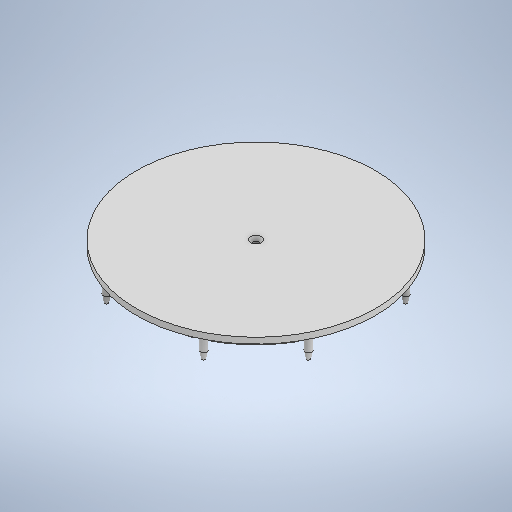
# Autodesk Inventor part: lid
Saved by Autodesk Inventor 2025 (Build 290162000, 162)
## iProperties
Created: 2026-05-09
Part Number: lid
Material: Generic
Document SubType Name: Modeling
Designer: Luca
Density: 1 g/cm^3
Appearance: Default
Author: Luca
Autodesk Inventor part; units mm, degrees
ref_plane "YZ Plane" through (0, 0, 0) normal (1, 0, 0) x (0, 1, 0)
ref_plane "XZ Plane" through (0, 0, 0) normal (0, 1, 0) x (-1, 0, 0)
ref_plane "XY Plane" through (0, 0, 0) normal (0, 0, 1) x (1, 0, 0)
sketch "lid" plane through (0, 0, 0) normal (0, 1, 0) x (-1, 0, 0)
  line L0 (35, 35) -> (-68.5857, 35)
  line L1 (38, 38) -> (-69.4029, 38)
  line L2 (80, 0) -> (-80, 0) construction
  circle A0 centre (0, 0) radius 80
  line L3 (0, -80) -> (0, 80) construction
  line L4 (38, -69.4029) -> (38, 38)
  line L5 (35, -68.5857) -> (35, 35)
  line L6 (0, 0) -> (56.5685, 56.5685) construction
  line L7 (36.5, 36.5) -> (36.5, -71.1881) construction
  line L8 (36.5, 36.5) -> (-71.1881, 36.5) construction
  line L9 (38, 38) -> (35, 35) construction
  line L10 (36.625, -71.1239) -> (36.625, 36.625)
  line L11 (36.375, 36.375) -> (36.375, -71.2521)
  line L12 (38, -69.4029) -> (38, -70.3989)
  line L13 (35, -68.5857) -> (35, -71.9375)
  line L14 (36.375, 36.375) -> (-71.2521, 36.375)
  line L15 (-71.1239, 36.625) -> (36.625, 36.625)
  line L16 (-69.4029, 38) -> (-70.3989, 38)
  line L17 (-68.5857, 35) -> (-71.9375, 35)
  line L18 (35, 34.8232) -> (56.6569, 56.4801)
  line L19 (32.8787, 35) -> (55.4979, 57.6193)
  line L20 (34.8232, 35) -> (56.4801, 56.6569)
  line L21 (35, 32.8787) -> (57.6193, 55.4979)
  line L22 (37.75, 37.75) -> (37.75, -70.5332)
  line L23 (35.25, -71.8153) -> (35.25, 35.25)
  line L24 (37.75, 37.75) -> (-70.5332, 37.75)
  line L25 (-71.8153, 35.25) -> (35.25, 35.25)
  line L26 (33.2322, 35) -> (55.6778, 57.4455)
  line L27 (57.4455, 55.6778) -> (35, 33.2322)
extrude "Extrusion1" add sketch "lid" along normal up to surface (4 mm away) from surface at 0
sketch "reservoir_lid_seal" plane through (0, 0, 0) normal (0, 1, 0) x (-1, 0, 0)
  line L0 (35, -68.5857) -> (35, 35) construction
  line L1 (35.25, -71.8153) -> (35.25, 35.25) construction
  line L2 (36.375, 36.375) -> (36.375, -71.2521) construction
  line L3 (36.5, 36.5) -> (36.5, -71.1881) construction
  line L4 (36.625, -71.1239) -> (36.625, 36.625) construction
  line L5 (37.75, 37.75) -> (37.75, -70.5332) construction
  line L6 (38, -69.4029) -> (38, 38) construction
  line L7 (0, -80) -> (0, 80) construction
  line L8 (80, 0) -> (-80, 0) construction
  line L9 (35, 35) -> (-68.5857, 35) construction
  line L10 (38, 38) -> (-69.4029, 38) construction
  line L11 (38, -69.4029) -> (38, -70.3989) construction
  line L12 (35, -68.5857) -> (35, -71.9375) construction
  line L13 (37.75, 37.75) -> (-70.5332, 37.75) construction
  line L14 (-71.1239, 36.625) -> (36.625, 36.625) construction
  line L15 (36.5, 36.5) -> (-71.1881, 36.5) construction
  line L16 (36.375, 36.375) -> (-71.2521, 36.375) construction
  line L17 (-71.8153, 35.25) -> (35.25, 35.25) construction
  line L18 (-69.4029, 38) -> (-70.3989, 38) construction
  line L19 (-68.5857, 35) -> (-71.9375, 35) construction
  line L20 (0, 0) -> (56.5685, 56.5685) construction
  line L21 (38, 38) -> (35, 35) construction
  line L22 (32.8787, 35) -> (55.4979, 57.6193)
  line L23 (33.2322, 35) -> (55.6778, 57.4455) construction
  line L24 (34.8232, 35) -> (56.4801, 56.6569) construction
  line L25 (35, 34.8232) -> (56.6569, 56.4801) construction
  line L26 (57.4455, 55.6778) -> (35, 33.2322) construction
  line L27 (35, 32.8787) -> (57.6193, 55.4979)
  circle A0 centre (-67.5925, 32.5) radius 2.2 construction
  circle A1 centre (-67.5925, 32.5) radius 2.5 construction
  circle A2 centre (-67.5925, 32.5) radius 5 construction
  line L28 (-67.5925, 32.5) -> (-67.5925, -32.5) construction
  circle A3 centre (-67.5925, -32.5) radius 2.2 construction
  circle A4 centre (-67.5925, -32.5) radius 2.5 construction
  circle A5 centre (-67.5925, -32.5) radius 5 construction
  line L29 (35, 35) -> (-68.5857, 35) construction
  line L30 (38, 38) -> (-69.4029, 38) construction
  circle A6 centre (-32.5, -67.5925) radius 5 construction
  line L31 (35, -68.5857) -> (35, 35) construction
  line L32 (38, -69.4029) -> (38, 38) construction
  circle A7 centre (0, 0) radius 80 construction
  line L33 (-32.5, -67.5925) -> (32.5, -67.5925) construction
  circle A8 centre (32.5, -67.5925) radius 5 construction
  circle A9 centre (-32.5, 67.5925) radius 2.2 construction
  circle A10 centre (-32.5, 67.5925) radius 2.5 construction
  circle A11 centre (67.5925, -32.5) radius 5 construction
  circle A12 centre (67.5925, 32.5) radius 2.2 construction
  circle A13 centre (67.5925, 32.5) radius 2.5 construction
  circle A14 centre (67.5925, 32.5) radius 5 construction
  line L34 (67.5925, 32.5) -> (67.5925, -32.5) construction
  circle A15 centre (67.5925, -32.5) radius 2.2 construction
  circle A16 centre (67.5925, -32.5) radius 2.5 construction
  circle A17 centre (-32.5, 67.5925) radius 5 construction
  circle A18 centre (32.5, 67.5925) radius 2.5 construction
  circle A19 centre (32.5, 67.5925) radius 5 construction
  line L35 (0, 67.5925) -> (0, 0) construction
  circle A20 centre (32.5, 67.5925) radius 2.2 construction
  line L36 (33.7759, 70.2462) -> (34.6667, 72.0987) construction
  line L37 (32.5, 67.5925) -> (-32.5, 67.5925) construction
  circle A21 centre (32.5, -67.5925) radius 2.5 construction
  circle A22 centre (-32.5, -67.5925) radius 2.5 construction
  circle A23 centre (32.5, -67.5925) radius 2.2 construction
  circle A24 centre (-32.5, -67.5925) radius 2.2 construction
  line L38 (67.5925, 0) -> (0, 0) construction
  line L39 (3.4, 0) -> (1.7, -2.9445) construction
  line L40 (1.7, 2.9445) -> (3.4, 0) construction
  line L41 (1.7, -2.9445) -> (-1.7, -2.9445) construction
  circle A25 centre (0, 0) radius 1.35 construction
  circle A26 centre (0, 0) radius 1.6 construction
  line L42 (-1.7, 2.9445) -> (1.7, 2.9445) construction
  line L43 (-1.7, -2.9445) -> (-3.4, 0) construction
  line L44 (-3.4, 0) -> (-1.7, 2.9445) construction
  circle A27 centre (0, 0) radius 5 construction
  circle A28 centre (67.5925, -32.5) radius 5.25
  circle A29 centre (32.5, -67.5925) radius 5.25
  circle A30 centre (-32.5, -67.5925) radius 5.25
  circle A31 centre (-67.5925, -32.5) radius 5.25
  circle A32 centre (-67.5925, 32.5) radius 5.25
  circle A33 centre (-32.5, 67.5925) radius 5.25
  circle A34 centre (32.5, 67.5925) radius 5.25
  circle A35 centre (67.5925, 32.5) radius 5.25
  circle A36 centre (0, 0) radius 5.25
  circle A37 centre (67.5925, -32.5) radius 6.25
  circle A38 centre (67.5925, 32.5) radius 6.25
  circle A39 centre (32.5, 67.5925) radius 6.25
  circle A40 centre (-32.5, 67.5925) radius 6.25
  circle A41 centre (-67.5925, 32.5) radius 6.25
  circle A42 centre (0, 0) radius 6.25
  circle A43 centre (-67.5925, -32.5) radius 6.25
  circle A44 centre (-32.5, -67.5925) radius 6.25
  circle A45 centre (32.5, -67.5925) radius 6.25
  line L45 (34.75, -72.0586) -> (34.75, 34.75)
  line L46 (34.75, 34.75) -> (-68.4324, 34.75)
  line L47 (-67.8159, 33.75) -> (33.75, 33.75)
  line L48 (33.75, 33.75) -> (33.75, -72.5323)
  arc A46 (38.25, -67.9775) -> (-67.9775, 38.25) centre (0, 0) ccw construction
  arc A47 (-68.5857, 35) -> (35, -68.5857) centre (0, 0) ccw construction
  arc A48 (-66.3253, 38.6202) -> (34.75, -68.4324) centre (0, 0) ccw
  arc A49 (-65.3373, 38.3289) -> (33.75, -67.8159) centre (0, 0) ccw
  arc A50 (38.25, -67.6905) -> (-67.6905, 38.25) centre (0, 0) ccw
  arc A51 (39.25, -65.9545) -> (-65.9545, 39.25) centre (0, 0) ccw
  line L49 (38.25, -67.6905) -> (38.25, 38.25)
  line L50 (38.25, 38.25) -> (-67.6905, 38.25)
  line L51 (-65.9545, 39.25) -> (39.25, 39.25)
  line L52 (39.25, 39.25) -> (39.25, -65.9545)
  point P0 (-67.5925, 0)
  point P1 (0, -67.5925)
  point P2 (-61.4688, 33.75)
  point P3 (33.75, -61.4688)
  point P4 (27.0986, -70.737)
  point P5 (-27.0986, -70.737)
  point P6 (-38.3289, -65.3373)
  point P7 (-65.3373, -38.3289)
  point P8 (-70.737, -27.0986)
  point P9 (-70.737, 27.0986)
  point P10 (-62.8491, 34.75)
  point P11 (-71.1911, 28.6773)
  point P12 (-71.1911, -28.6773)
  point P13 (-66.8539, -37.6978)
  point P14 (-37.6978, -66.8539)
  point P15 (-28.6773, -71.1911)
  point P16 (28.6773, -71.1911)
  point P17 (34.75, -62.8491)
  point P18 (37.7358, 67.9785)
  point P19 (29.532, 71.923)
  point P20 (-29.532, 71.923)
  point P21 (-37.7358, 67.9785)
  point P22 (-67.4071, 38.7472)
  point P23 (-65.143, 38.25)
  point P24 (67.9785, -37.7358)
  point P25 (71.923, -29.532)
  point P26 (71.923, 29.532)
  point P27 (67.9785, 37.7358)
  point P28 (66.3253, 38.6202)
  point P29 (71.5815, 27.6885)
  point P30 (71.5815, -27.6885)
  point P31 (66.3253, -38.6202)
  point P32 (-38.6202, 66.3253)
  point P33 (-27.6885, 71.5815)
  point P34 (27.6885, 71.5815)
  point P35 (38.6202, 66.3253)
extrude "Extrusion2" add sketch "reservoir_lid_seal" against normal blind 2 contours L50 A41 A50 A40 A51 L51 L22 | L22 L51 L52 L27 L49 L50 | A51 A39 A50 L22 | L22 A50 L27 A51 | L27 L52 A51 A37 A50 A45 L49 | L46 L45 A45 L48 L47 A41 | A41 L47 A32 L46 | L27 A50 A38 A51 | A51 A34 A50 A39 | A39 A51 A34 | A51 A33 A40 | A40 A50 A33 A51 | A45 A50 L49 | A41 A49 A32 L47 | A51 A35 A38 | A38 A50 A35 A51 | A51 A40 A50 A39 | A39 A50 A34 A51 | L45 A29 L48 A45 | A51 A35 A50 A38 | A38 A50 A37 A51 | A51 A33 A50 A40 | A51 A28 A50 A37 | A37 A51 A28 | L48 A29 A49 A45 | A49 A43 A48 A41 | A41 A48 A32 A49 | A37 A50 A28 A51 | A48 A44 A49 A45 | A45 A49 A29 A48 | A49 A31 A48 A43 | A43 A49 A31 | A48 A30 A49 A44 | A49 A30 A44 | A48 A31 A49 A43 | A43 A49 A44 A48 | A44 A49 A30 A48 | A42
sketch "lid_mount" plane through (0, -70, 0) normal (0, 1, 0) x (-1, 0, 0)
  line L0 (35, -68.5857) -> (35, 35) construction
  line L1 (35, 35) -> (-68.5857, 35) construction
  line L2 (38, 38) -> (-69.4029, 38) construction
  line L3 (38, -69.4029) -> (38, 38) construction
  circle A0 centre (32.5, -67.5925) radius 5
  circle A1 centre (-67.5925, 32.5) radius 5
  circle A2 centre (-67.5925, -32.5) radius 5
  circle A3 centre (-32.5, -67.5925) radius 5
  line L4 (-32.5, -67.5925) -> (32.5, -67.5925) construction
  circle A4 centre (0, 0) radius 80
  circle A5 centre (-67.5925, -32.5) radius 2.5
  circle A6 centre (32.5, -67.5925) radius 2.5
  circle A7 centre (-67.5925, 32.5) radius 2.5
  circle A8 centre (-32.5, -67.5925) radius 2.5
  circle A9 centre (67.5925, -32.5) radius 5
  circle A10 centre (-32.5, 67.5925) radius 5
  circle A11 centre (67.5925, -32.5) radius 2.5
  circle A12 centre (-32.5, 67.5925) radius 2.5
  circle A13 centre (32.5, 67.5925) radius 2.5
  circle A14 centre (32.5, 67.5925) radius 5
  circle A15 centre (67.5925, 32.5) radius 2.5
  circle A16 centre (67.5925, 32.5) radius 5
  line L5 (67.5925, 32.5) -> (67.5925, -32.5) construction
  line L6 (32.5, 67.5925) -> (-32.5, 67.5925) construction
  line L7 (0, 67.5925) -> (0, 0)
  line L8 (67.5925, 0) -> (0, 0)
  circle A17 centre (-67.5925, -32.5) radius 2.2
  circle A18 centre (32.5, 67.5925) radius 2.2
  circle A19 centre (67.5925, 32.5) radius 2.2
  circle A20 centre (32.5, -67.5925) radius 2.2
  circle A21 centre (-32.5, -67.5925) radius 2.2
  circle A22 centre (-67.5925, 32.5) radius 2.2
  circle A23 centre (-32.5, 67.5925) radius 2.2
  line L9 (33.7759, 70.2462) -> (34.6667, 72.0987) construction
  circle A24 centre (67.5925, -32.5) radius 2.2
  circle A25 centre (0, 0) radius 1.6
  line L10 (-3.4, 0) -> (-1.7, 2.9445)
  line L11 (-1.7, 2.9445) -> (1.7, 2.9445)
  line L12 (1.7, 2.9445) -> (3.4, 0)
  line L13 (3.4, 0) -> (1.7, -2.9445)
  line L14 (1.7, -2.9445) -> (-1.7, -2.9445)
  line L15 (-1.7, -2.9445) -> (-3.4, 0)
  circle A26 centre (0, 0) radius 5
  circle A27 centre (0, 0) radius 1.35
  line L16 (-67.5925, 32.5) -> (-67.5925, -32.5) construction
  point P0 (0, -67.5925)
  point P1 (-67.5925, 0)
extrude "Extrusion3" cut sketch "lid_mount" along normal through all contours A25 L8 A27 L7 | L7 A27 L8 A25 | A27 L8 L7 | L7 L8 A27
extrude "Extrusion4" add sketch "lid_mount" against normal blind 15 from surface at 70 contours A17 | A18 | A19 | A20 | A21 | A22 | A23 | A24
chamfer "Chamfer1" distance 1 distance2 5 1 edges at (34.7, -15, 67.5925) measured on face at (34.2, -15, 67.5925)
chamfer "Chamfer2" distance 1 distance2 5 1 edges at (-30.3, -15, 67.5925) measured on face at (-30.8, -15, 67.5925)
chamfer "Chamfer3" distance 1 distance2 5 1 edges at (-65.3925, -15, 32.5) measured on face at (-65.8925, -15, 32.5)
chamfer "Chamfer4" distance 1 distance2 5 1 edges at (-65.3925, -15, -32.5) measured on face at (-65.8925, -15, -32.5)
chamfer "Chamfer5" distance 1 distance2 5 1 edges at (-30.3, -15, -67.5925) measured on face at (-30.8, -15, -67.5925)
chamfer "Chamfer6" distance 1 distance2 5 1 edges at (34.7, -15, -67.5925) measured on face at (34.2, -15, -67.5925)
chamfer "Chamfer7" distance 1 distance2 5 1 edges at (69.7925, -15, -32.5) measured on face at (69.2925, -15, -32.5)
chamfer "Chamfer8" distance 1 distance2 5 1 edges at (69.7925, -15, 32.5) measured on face at (69.2925, -15, 32.5)
sketch "pipe_out" plane through (-77.5, 0, 0) normal (1, 0, 0) x (0, 1, 0)
  line L0 (-132, 0) -> (302, 0)
  circle A0 centre (-10, 0) radius 7.5
  line L1 (0, 153.4424) -> (0, -148.4939)
  circle A1 centre (-10, 0) radius 7.25
  circle A2 centre (-10, 0) radius 5
  circle A3 centre (-10, 0) radius 9.5
  circle A4 centre (-10, 0) radius 6
  circle A5 centre (-10, 0) radius 6.25
  circle A6 centre (-10, 0) radius 9.75
  point P0 (0, 0)
  point P1 (-2.5, 0)
  point P2 (-2.75, 0)
extrude "Extrusion5" cut sketch "pipe_out" along normal mid plane 10
sketch "battery_lid" plane through (0, -57.9, 0) normal (0, 1, 0) x (-1, 0, 0)
  arc A0 (38.25, -67.9775) -> (-67.9775, 38.25) centre (0, 0) ccw construction
  line L0 (0, -80) -> (0, 80) construction
  circle A1 centre (0, 0) radius 80
  arc A2 (-14.9031, 77.5816) -> (-20.7481, 76.2267) centre (0, 0) ccw
  arc A3 (-14.2257, 74.659) -> (-20.0707, 73.3042) centre (0, 0) ccw
  line L1 (-17.1615, 74.0393) -> (-17.8385, 76.9597) construction
  line L2 (-14.9031, 77.5816) -> (-14.2257, 74.659)
  line L3 (-20.0707, 73.3042) -> (-20.7481, 76.2267)
  arc A4 (20.2646, 72.9914) -> (-20.2646, 72.9914) centre (0, 0) ccw
  line L4 (20.2646, 72.9914) -> (21.4009, 77.0844) construction
  line L5 (-20.2646, 72.9914) -> (-21.4009, 77.0844) construction
  line L6 (-14.5278, 74.8555) -> (-15.0922, 77.2903)
  line L7 (-19.8858, 73.6136) -> (-20.4501, 76.0484)
  arc A5 (-14.5278, 74.8555) -> (-19.8858, 73.6136) centre (0, 0) ccw
  arc A6 (-15.0922, 77.2903) -> (-20.4501, 76.0484) centre (0, 0) ccw
  line L8 (25, 80) -> (-25, 80) construction
  line L9 (14.5278, 74.8555) -> (15.0922, 77.2903)
  arc A7 (20.4501, 76.0484) -> (15.0922, 77.2903) centre (0, 0) ccw
  line L10 (19.8858, 73.6136) -> (20.4501, 76.0484)
  arc A8 (19.8858, 73.6136) -> (14.5278, 74.8555) centre (0, 0) ccw
  arc A9 (20.7481, 76.2267) -> (14.9031, 77.5816) centre (0, 0) ccw
  line L11 (17.1615, 74.0393) -> (17.8385, 76.9597) construction
  arc A10 (20.0707, 73.3042) -> (14.2257, 74.659) centre (0, 0) ccw
  line L12 (20.0707, 73.3042) -> (20.7481, 76.2267)
  line L13 (14.9031, 77.5816) -> (14.2257, 74.659)
  line L14 (-27.5, 72.9914) -> (-20.2646, 72.9914)
  line L15 (20.2646, 72.9914) -> (27.5, 72.9914)
  arc A11 (-4.983, 75.5882) -> (4.983, 75.5882) centre (0, 76) ccw
  circle A12 centre (0, 76) radius 3
  arc A13 (12.7529, 78.977) -> (-12.7529, 78.977) centre (0, 71.0799) ccw
  line L16 (-29.5024, 73.2792) -> (-29.8776, 74.2114)
  line L17 (29.5024, 73.2792) -> (29.8776, 74.2114)
  line L18 (27.879, 73.9328) -> (27.5, 72.9914)
  line L19 (-27.879, 73.9328) -> (-27.5, 72.9914)
  line L20 (-28.0175, 73.6075) -> (-27.6688, 72.7414)
  line L21 (28.0175, 73.6075) -> (27.6688, 72.7414)
  line L22 (29.6409, 72.9539) -> (30.1094, 74.1176)
  line L23 (-29.6409, 72.9539) -> (-30.1094, 74.1176)
  line L24 (-20.0936, 71.7414) -> (-28.3442, 71.7414)
  line L25 (28.3442, 71.7414) -> (20.0936, 71.7414)
  arc A14 (-5.2061, 75.3225) -> (5.2061, 75.3225) centre (0, 76) ccw
  line L26 (31.0336, 73.7355) -> (30.1951, 71.6528)
  line L27 (30.1951, 71.6528) -> (28.5717, 72.3064)
  line L28 (-31.0336, 73.7355) -> (-30.1951, 71.6528)
  line L29 (-30.1951, 71.6528) -> (-28.5717, 72.3064)
  line L30 (-28.5717, 72.3064) -> (-28.3442, 71.7414)
  line L31 (28.5717, 72.3064) -> (28.3442, 71.7414)
  line L32 (-29.5024, 73.2792) -> (-27.879, 73.9328)
  line L33 (-29.6409, 72.9539) -> (-28.0175, 73.6075)
  line L34 (-29.0642, 74.5337) -> (-28.3172, 72.6783) construction
  line L35 (29.0642, 74.5337) -> (28.3172, 72.6783) construction
  line L36 (28.0175, 73.6075) -> (29.6409, 72.9539)
  line L37 (29.5024, 73.2792) -> (27.879, 73.9328)
  arc A15 (20.2305, 72.7414) -> (-20.2305, 72.7414) centre (0, 0) ccw
  line L38 (27.6688, 72.7414) -> (20.2305, 72.7414)
  line L39 (-27.6688, 72.7414) -> (-20.2305, 72.7414)
  line L40 (28.5717, 72.3064) -> (27.4912, 72.7414)
  line L41 (-28.5717, 72.3064) -> (-27.4912, 72.7414)
  arc A16 (20.0936, 71.7414) -> (-20.0936, 71.7414) centre (0, 0) ccw
  line L42 (28.5717, 72.3064) -> (28.9452, 73.234)
  line L43 (-28.5717, 72.3064) -> (-28.9452, 73.234)
  line L44 (38.25, 38.25) -> (-68.9797, 38.25) construction
  line L45 (-26.75, 38.25) -> (-26.75, 55.25)
  line L46 (-26.75, 55.25) -> (26.75, 55.25)
  line L47 (26.75, 55.25) -> (26.75, 38.25)
  line L48 (-26.75, 38.25) -> (26.75, 38.25)
  line L49 (-26.5, 38.5) -> (-26.5, 55)
  line L50 (-26.5, 55) -> (26.5, 55)
  line L51 (26.5, 55) -> (26.5, 38.5)
  line L52 (26.5, 38.5) -> (-26.5, 38.5)
  arc A17 (-6.2045, 75.2469) -> (6.2045, 75.2469) centre (0, 76) ccw
  line L53 (3, 76) -> (3, 79)
  line L54 (3, 79) -> (-3, 79)
  line L55 (-3, 79) -> (-3, 76)
  point P0 (-25, 80)
  point P1 (25, 80)
  point P2 (-17.5, 75.4995)
  point P3 (17.5, 75.4995)
  point P4 (17.5, 75.4995)
  point P5 (-28.6907, 73.606)
  point P6 (28.6907, 73.606)
  point P7 (0, 0)
  point P8 (-26.5, 80)
  point P9 (-26.5, 80)
  point P10 (-26.5, 80)
  point P11 (26.5, 80)
  point P12 (26.5, 80)
  point P13 (26.5, 80)
  point P14 (-2.9843, 75.6934)
  point P15 (2.9843, 75.6934)
  point P16 (-6.0029, 74.26)
  point P17 (6.0029, 74.26)
  point P18 (4.9562, 75.3394)
  point P19 (-4.9562, 75.3394)
extrude "Extrusion6" cut sketch "battery_lid" against normal blind 10 from surface at 57.9 contours L26 L27 L42 L36 L22 A1 | A1 L23 L33 L43 L29 L28 | L22 L36 L21 L38 A15 A11 A4 L15 L18 L37 L17 A1 | A1 L16 L32 L19 L14 A4 A11 A15 L39 L20 L33 L23 | L17 L37 L18 L15 A4 A12 L53 L54 L55 L14 L19 L32 L16 A1 | L40 L38 L21 L36 L42 | L43 L33 L20 L39 L41 | A4 A12 | A12 L54 L53 | L55 L54 A12 | L2 A3 L3 A2 | A5 L7 A6 L6 | L9 A7 L10 A8 | L12 A10 L13 A9
extrude "Extrusion7" add sketch "battery_lid" against normal blind 2 from surface at 57.9 contours L31 L25 A16 A17 A15 L38 L40 | L41 L39 A15 A17 A16 L24 L30 | A17 A16 A14 | A16 A14 A15 A17 | A17 A15 A14 A16
extrude "Extrusion8" cut sketch "battery_lid" along normal mid plane 2.5 from surface at 59.9 contours A12 A15 A4 | A4 A12 | A16 A12 A15 | A12 A16 | A12 L54 L53 | L55 L54 A12
fillet "Fillet1" radius 8.75 2 edges at (6.0029, -1, 74.26) (-6.0029, -1, 74.26)
fillet "Fillet2" radius 9.75 2 edges at (5.2061, -1, 75.3225) (-5.2061, -1, 75.3225)
chamfer "Chamfer9" distance 2 angle 45 1 edges at (1.6, 4, 0)
body "Solid1"
